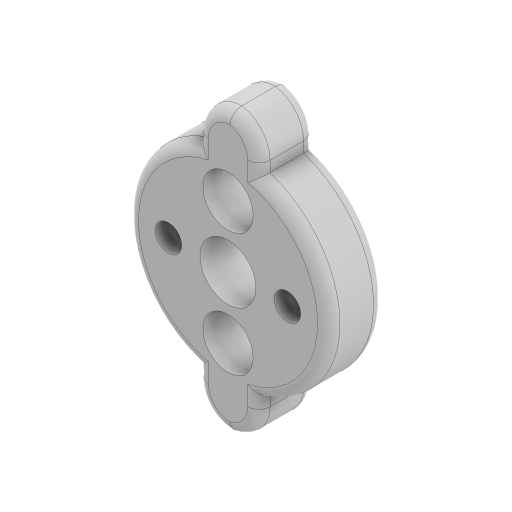
# Autodesk Inventor part: turning_cap
Saved by Autodesk Inventor 2024 (Build 280153000, 153)
## iProperties
Created: 2024-07-08
Part Number: turning_cap
Material: Generic
Document SubType Name: Modeling
Designer: chris
Density: 1 g/cm^3
Appearance: Default
Author: chris
Autodesk Inventor part; units mm, degrees
ref_plane "YZ Plane" through (0, 0, 0) normal (1, 0, 0) x (0, 1, 0)
ref_plane "XZ Plane" through (0, 0, 0) normal (0, 1, 0) x (-1, 0, 0)
ref_plane "XY Plane" through (0, 0, 0) normal (0, 0, 1) x (1, 0, 0)
sketch "Sketch1" plane through (0, 0, 0) normal (0, 0, 1) x (1, 0, 0)
  circle A0 centre (0, 0) radius 11.43
  circle A1 centre (-6.75, 0) radius 1.5
  circle A2 centre (0, 0) radius 1.5
  circle A3 centre (6.75, 0) radius 1.5
  line L0 (0, 0) -> (0, 6.985)
  line L1 (0, 0) -> (0, -6.985)
  circle A4 centre (0, 6.985) radius 1.4986
  circle A5 centre (0, -6.985) radius 1.4986
  circle A6 centre (0, 0) radius 3.175
  arc A7 (0.31, -15.875) -> (3.5, -12.1158) centre (-0.31, -12.1158) ccw
  line L2 (3.5, -12.1158) -> (3.5, 12.1158)
  arc A8 (3.5, 12.1158) -> (0.31, 15.875) centre (-0.31, 12.1158) ccw
  arc A9 (0.31, 15.875) -> (-3.5, 12.065) centre (0.31, 12.065) ccw
  line L3 (-3.5, 12.065) -> (-3.5, -12.065)
  arc A10 (-3.5, -12.065) -> (0.31, -15.875) centre (0.31, -12.065) ccw
  circle A11 centre (0, 6.985) radius 1.5
  circle A12 centre (0, -6.985) radius 1.5
  line L4 (3.5, 0) -> (-3.5, 0)
  line L5 (0, 0) -> (0, 6.985)
  point P0 (3.5, -10.8809)
  point P1 (-3.5, -10.8809)
  point P2 (-3.5, 10.8809)
  point P3 (3.5, 10.8809)
  dimension "d0" = 22.86
  dimension "d1" = 6.985
  dimension "d2" = 6.985
  dimension "d3" = 2.9972
  dimension "d4" = 2.9972
  dimension "d7" = 6.35
  constraints: 13 centre point, 12 end point, 8 point on circle, 4 coincident, 2 midpoint, 2 vertical
  measures "d0" diameter of A0
  measures "d1" distance of L0.start L0.end
  measures "d2" distance of L0.start L1.end
  measures "d3" diameter of A4
  measures "d4" diameter of A5
  measures "d7" diameter of A6
extrude "Extrusion1" add sketch "Sketch1" along normal blind 6.35 contours A0 L2 | L2 L4 A6 L3 A0 | A0 L3 A9 A8 L2 | L2 A7 A10 L3 A0 | A0 L3 L4 A6 L2 | L3 A0
fillet "Fillet2" radius 1.27 20 edges at (11.43, 0, 0) (11.43, 0, 6.35) (-11.43, 0, 0) (-11.43, 0, 6.35) (3.5, 11.4984, 6.35) (2.595, 14.5809, 6.35) (-3.5, 11.473, 6.35) (-2.3841, 14.7591, 6.35) (-3.5, 11.473, 0) (-2.3841, 14.7591, 0) (3.5, 11.4984, 0) (2.595, 14.5809, 0) (2.595, -14.5809, 6.35) (3.5, -11.4984, 6.35) (-3.5, -11.473, 6.35) (-2.3841, -14.7591, 6.35) (3.5, -11.4984, 0) (2.595, -14.5809, 0) (-3.5, -11.473, 0) (-2.3841, -14.7591, 0)
sketch "Sketch3" plane through (0, 0, 6.35) normal (0, 0, 1) x (1, 0, 0)
  circle A0 centre (0, 6.985) radius 1.4986 projected
  circle A1 centre (0, 6.985) radius 2.8575
  circle A2 centre (0, -6.985) radius 1.4986 projected
  circle A3 centre (0, -6.985) radius 2.8575
  point P0 (0, 0)
  dimension "d12" = 5.715
  dimension "d13" = 5.715
  constraints: 2 centre point, 2 coincident
  measures "d12" diameter of A1
  measures "d13" diameter of A3
extrude "Extrusion2" cut sketch "Sketch3" against normal blind 4.7625
body "Solid1"
